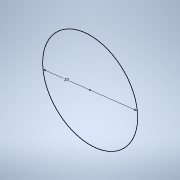
# Autodesk Inventor part: embudo
Saved by Autodesk Inventor 2020.3 (Build 243373000, 373)
## iProperties
Created: 2021-02-17
Part Number: embudo
Material: Generic
Document SubType Name: Modeling
Designer: juanp
Density: 1 g/cm^3
Appearance: Default
Author: juanp
Autodesk Inventor part; units mm, degrees
ref_plane "YZ Plane" through (0, 0, 0) normal (1, 0, 0) x (0, 1, 0)
ref_plane "XZ Plane" through (0, 0, 0) normal (0, 1, 0) x (-1, 0, 0)
ref_plane "XY Plane" through (0, 0, 0) normal (0, 0, 1) x (1, 0, 0)
sketch "Sketch1" plane through (0, 0, 0) normal (0, 0, 1) x (1, 0, 0)
  line L0 (-37.5, 75) -> (-10, 11.8427)
  line L1 (37.5, 75) -> (10, 11.8427)
  arc A0 (-10, 11.8427) -> (-10, -11.8427) centre (0, 0) ccw
  arc A1 (10, -11.8427) -> (10, 11.8427) centre (0, 0) ccw
  line L2 (-10, -11.8427) -> (-5, -20)
  line L3 (10, -11.8427) -> (5, -20)
  line L4 (-5, -20) -> (5, -20)
  circle A2 centre (0, 0) radius 5.5
  line L5 (0, 0) -> (0, -20) construction
  line L6 (37.5, 75) -> (-37.5, 75)
  line L7 (0, 75) -> (0, 0) construction
  line L8 (39.6814, 75) -> (-39.6814, 75)
  line L9 (-39.6814, 75) -> (-12.4012, 12.3475)
  arc A3 (-12.4012, 12.3475) -> (-11.5419, -13.1543) centre (0, 0) ccw
  line L10 (-11.5419, -13.1543) -> (-7.3458, -20)
  line L11 (7.3458, -20) -> (11.5419, -13.1543)
  line L12 (12.4012, 12.3475) -> (39.6814, 75)
  arc A4 (11.5419, -13.1543) -> (12.4012, 12.3475) centre (0, 0) ccw
  line L13 (7.3458, -20) -> (-7.3458, -20)
  point P0 (-37.5, 75)
  dimension "d1" = 15.5
  dimension "d2" = 10
  dimension "d3" = 11
  dimension "d4" = 75
  dimension "d5" = 20
  dimension "d6" = 20
  dimension "d7" = 20
  dimension "d8" = 75
  dimension "d9" = 2
  dimension "d10" = 2
  dimension "d11" = 2
  constraints: 28 end point, 8 point on circle, 5 centre point, 4 concentric, 4 equal length, 4 parallel, 3 coincident, 3 collinear, 3 horizontal, 2 midpoint, 2 vertical
  measures "d1" radius of A1
  measures "d2" distance of L3.end L2.end
  measures "d3" diameter of A2
  measures "d4" distance of L1.start L0.start
  measures "d5" distance of L0.end L1.end
  measures "d6" distance of L2.start L3.start
  measures "d7" distance from line of point (0, 0) L4
  measures "d8" distance from line of L6 point (0, 0)
  measures "d9" radial gap between concentric circles of A0 A3
  measures "d10" distance between parallel lines of L2 L10
  measures "d11" distance between parallel lines of L0 L9
extrude "Extrusion1" add sketch "Sketch1" against normal blind 2
extrude "Extrusion2" add sketch "Sketch1" along normal blind 20 contours L0 A0 L2 L13 L10 A3 L9 L8 | L8 L12 A4 L11 L13 L3 A1 L1
ref_plane "Work Plane1" through (0, 0, 10) normal (0, 0, 1) x (1, 0, 0)
mirror "Mirror1" about plane through (0, 0, 10) normal (0, 0, 1) of "Extrusion1"
sketch "Sketch3" plane through (-39.6814, 75, 22) normal (0, 0, 1) x (1, 0, 0)
  line L0 (39.6814, -75) -> (39.6814, -60.389) construction
  line L1 (34.7564, -60.389) -> (44.6064, -60.389) construction
  circle A0 centre (34.7564, -60.389) radius 0.75
  circle A1 centre (44.6064, -60.389) radius 0.75
  circle A2 centre (34.7564, -60.389) radius 3.75
  circle A3 centre (44.6064, -60.389) radius 3.75
  dimension "d17" = 14.611
  dimension "d18" = 9.85
  dimension "d19" = 1.5
  dimension "d20" = 3
  dimension "d21" = 3
  constraints: 4 centre point, 4 coincident, 4 end point, 1 equal radius, 1 horizontal, 1 midpoint, 1 vertical
  measures "d17" distance of L0.end L0.start
  measures "d18" distance of L1.start L1.end
  measures "d19" diameter of A1
  measures "d20" radial gap between concentric circles of A2 A0
  measures "d21" radial gap between concentric circles of A3 A1
extrude "Extrusion3" add sketch "Sketch3" along normal blind 11.9
chamfer "Chamfer1" distance 2 angle 45 2 edges at (-8.675, 14.611, 22) (1.175, 14.611, 22)
ref_plane "Work Plane2" through (37.5, 75, 20) normal (0, 0, -1) x (-1, 0, 0)
split body "Split1" result two bodies by plane through (37.5, 75, 20) normal (0, 0, -1) first body at (-4.1337, 54.1158, -1.5)
sketch "Sketch4" plane through (37.5, 75, 20) normal (0, 0, -1) x (-1, 0, 0)
  circle A0 centre (37.5, -75) radius 5.5 projected
  line L0 (-2.1814, 0) -> (77.1814, 0) projected
  line L1 (25.0988, -62.6525) -> (-2.1814, 0) projected
  arc A1 (25.0988, -62.6525) -> (25.9581, -88.1543) centre (37.5, -75) ccw projected
  line L2 (30.1542, -95) -> (25.9581, -88.1543) projected
  line L3 (44.8458, -95) -> (30.1542, -95) projected
  line L4 (49.0419, -88.1543) -> (44.8458, -95) projected
  arc A2 (49.0419, -88.1543) -> (49.9012, -62.6525) centre (37.5, -75) ccw projected
  line L5 (77.1814, 0) -> (49.9012, -62.6525) projected
  line L6 (-2.1814, 0) -> (25.0988, -62.6525) projected
  line L7 (-2.1814, 0) -> (-3.2721, 0)
  line L8 (-3.2721, 0) -> (23.9161, -62.441)
  line L9 (49.9012, -62.6525) -> (77.1814, 0) projected
  line L10 (77.1814, 0) -> (78.2721, 0)
  line L11 (78.2721, 0) -> (51.0839, -62.441)
  arc A3 (23.9161, -62.441) -> (24.4917, -88.1543) centre (37.5, -75) ccw
  arc A4 (50.5083, -88.1543) -> (51.0839, -62.441) centre (37.5, -75) ccw
  arc A5 (49.0419, -88.1543) -> (49.9012, -62.6525) centre (37.5, -75) ccw projected
  arc A6 (25.0988, -62.6525) -> (25.9581, -88.1543) centre (37.5, -75) ccw projected
  arc A7 (49.0419, -88.1543) -> (49.9012, -62.6525) centre (37.5, -75) ccw projected
  line L12 (49.0419, -88.1543) -> (50.5083, -88.1543)
  line L13 (24.4917, -88.1543) -> (25.9581, -88.1543)
  dimension "d28" = 1
  dimension "d29" = 1
  constraints: 13 end point, 4 horizontal, 4 point on circle, 3 concentric, 2 centre point, 2 parallel, 1 equal length
  measures "d28" distance between parallel lines of L1 L8
  measures "d29" radial gap between concentric circles of A3 A1
extrude "Extrusion4" add sketch "Sketch4" against normal mid plane 4 contours L1 A1 L13 A3 L8 L7 | L10 L11 A4 L12 A2 L5 bodies 2
chamfer "Chamfer2" distance 1 angle 45 4 edges at (17.4901, -0.5893, 18) (26.0413, 43.6738, 18) (-17.4901, -0.5893, 18) (-26.0413, 43.6738, 18)
body "Solid2"
body "Solid3"
